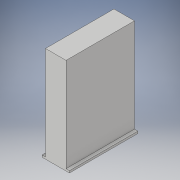
# Autodesk Inventor part: Netgear Router
Saved by Autodesk Inventor 2018 (Build 220112000, 112)
## iProperties
Created: 2019-01-10
Part Number: Netgear Router
Material: Generic
Document SubType Name: Modeling
Designer: snipe
Density: 1 g/cm^3
Appearance: Default
Author: snipe
Autodesk Inventor part; units mm, degrees
ref_plane "YZ Plane" through (0, 0, 0) normal (1, 0, 0) x (0, 1, 0)
ref_plane "XZ Plane" through (0, 0, 0) normal (0, 1, 0) x (-1, 0, 0)
ref_plane "XY Plane" through (0, 0, 0) normal (0, 0, 1) x (1, 0, 0)
sketch "Sketch1" plane through (0, 0, 0) normal (0, 1, 0) x (-1, 0, 0)
  line L0 (0, -88.9) -> (0, 88.9) projected
  line L1 (-26.67, 0) -> (26.67, 0) projected
  line L2 (26.67, 0) -> (-26.67, 0) projected
  line L3 (0, -88.9) -> (0, 88.9) projected
  line L4 (19.05, 63.5) -> (-19.05, 63.5)
  line L5 (-19.05, 63.5) -> (-19.05, -63.5)
  line L6 (-19.05, -63.5) -> (19.05, -63.5)
  line L7 (19.05, -63.5) -> (19.05, 63.5)
  line L8 (19.05, 63.5) -> (-19.05, -63.5) construction
  line L9 (-19.05, 63.5) -> (19.05, -63.5) construction
  point P0 (0, 0)
  dimension "d0" = 38.1
  dimension "d1" = 127
  constraints: 12 end point, 2 midpoint, 2 parallel, 1 horizontal, 1 perpendicular
  measures "d0" distance of L6.end L5.end
  measures "d1" distance of L5.end L4.end
extrude "Extrusion1" add sketch "Sketch1" along normal blind 177.8
sketch "Sketch2" plane through (0, 0, 0) normal (0, -1, 0) x (1, 0, 0)
  line L0 (-25.4, -63.5) -> (25.4, -63.5)
  line L1 (25.4, -63.5) -> (25.4, 63.5)
  line L2 (25.4, 63.5) -> (-25.4, 63.5)
  line L3 (-25.4, 63.5) -> (-25.4, -63.5)
  line L4 (-25.4, -63.5) -> (25.4, 63.5) construction
  line L5 (25.4, -63.5) -> (-25.4, 63.5) construction
  point P0 (0, 0)
  dimension "d4" = 50.8
  constraints: 12 end point, 2 midpoint, 2 parallel, 1 horizontal, 1 perpendicular
  measures "d4" distance of L2.end L1.end
extrude "Extrusion2" add sketch "Sketch2" against normal blind 3.81
body "Solid1"
